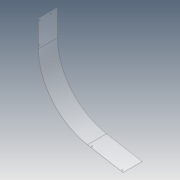
# Autodesk Inventor part: GE-12070-02
Saved by Autodesk Inventor 2012 (Build 160160000, 160)
## iProperties
Created: 2011-09-22
Part Number: GE-12070-02
Document SubType Name: Modeling
Designer: dfoster
Density: 1 g/cm^3
Description: Front
Material: Default
Title: Front
Author: dfoster
Autodesk Inventor part; units mm, degrees
ref_plane "YZ Plane" through (0, 0, 0) normal (1, 0, 0) x (0, 1, 0)
ref_plane "XZ Plane" through (0, 0, 0) normal (0, 1, 0) x (-1, 0, 0)
ref_plane "XY Plane" through (0, 0, 0) normal (0, 0, 1) x (1, 0, 0)
sketch "Sketch1" plane through (0, 0, 0) normal (0, 0, 1) x (1, 0, 0)
  line L0 (386.5124, -118.4812) -> (167.8098, -79.9181) projected
  arc A0 (-132.6001, 278.0965) -> (167.8098, -79.9181) centre (230.9374, 278.0965) ccw projected
  line L1 (-132.6001, 278.0965) -> (-132.6001, 439.2052) projected
  line L2 (-135.7751, 439.2052) -> (-132.6001, 439.2052) projected
  line L3 (-135.7751, 439.2052) -> (-135.7751, 278.0965) projected
  arc A1 (-135.7751, 278.0965) -> (167.2585, -83.0448) centre (230.9374, 278.0965) ccw projected
  line L4 (167.2585, -83.0448) -> (386.5124, -121.7052) projected
  line L5 (386.5124, -118.4812) -> (386.5124, -121.7052) projected
  point P0 (0, 0)
extrude "Extrusion1" add sketch "Sketch1" along normal blind 117.475
hole "Hole1" at (-132.6001, 426.5052, 109.5375) direction (-1, 0, 0) diameter 6.731 depth 25.4 tip angle 118
pattern_linear "Rectangular Pattern1" count 2 spacing 68.2625 along (0, 0, -1) of "Hole1"
pattern_linear "Rectangular Pattern2" count 2 spacing 133.35 along (0, -1, 0) of "Hole1"
hole "Hole2" at (374.0054, -119.4999, 109.5375) direction (0.1736, 0.9848, 0) diameter 6.731 depth 25.4 tip angle 118
pattern_linear "Rectangular Pattern4" count 2 spacing 190.5 along (-0.9848, 0.1736, 0) of "Hole2"
body "Solid1"
